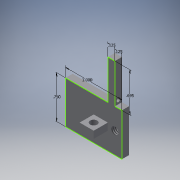
# Autodesk Inventor part: slide pivot plate
Saved by Autodesk Inventor 2016 (Build 200138000, 138)
## iProperties
Created: 2017-01-31
Part Number: slide pivot plate
Material: Generic
Document SubType Name: Modeling
Designer: Mark Koeppen
Density: 1 g/cm^3
Appearance: Default
Mass: 1.61101 g
Surface Area: 14.7029 cm^2
Volume: 1.61101 cm^3
Author: Mark Koeppen
Autodesk Inventor part; units mm, degrees
ref_plane "YZ Plane" through (0, 0, 0) normal (1, 0, 0) x (0, 1, 0)
ref_plane "XZ Plane" through (0, 0, 0) normal (0, 1, 0) x (-1, 0, 0)
ref_plane "XY Plane" through (0, 0, 0) normal (0, 0, 1) x (1, 0, 0)
sketch "Sketch1" plane through (0, 0, 0) normal (0, 0, 1) x (1, 0, 0)
  line L0 (0, -21.016) -> (25.4, -21.016)
  line L1 (25.4, -21.016) -> (25.4, -1.966)
  line L2 (0, -1.966) -> (0, -21.016)
  line L3 (19.05, -1.966) -> (19.05, 15.687)
  line L4 (19.05, 15.687) -> (22.225, 15.687)
  line L5 (22.225, 15.687) -> (22.225, -1.966)
  line L6 (25.4, -1.966) -> (22.225, -1.966)
  line L7 (19.05, -1.966) -> (0, -1.966)
  dimension "d0" = 19.05
  dimension "d2" = 25.4
  dimension "d3" = 3.175
  dimension "d4" = 17.653
  dimension "d22" = 3.175
  constraints: 16 end point, 4 parallel, 4 perpendicular, 1 collinear, 1 horizontal
  measures "d0" distance of L2.start L0.start
  measures "d2" distance of L1.end L2.start
  measures "d3" distance between parallel lines of L5 L3
  measures "d4" distance between parallel lines of L6 L4
  measures "d22" distance between parallel lines of L5 L1
extrude "Extrusion1" add sketch "Sketch1" against normal blind 3.175
sketch "Sketch2" plane through (0, 0, 0) normal (0, 0, 1) x (1, 0, 0)
  line L0 (12.7, -13.0785) -> (19.05, -13.0785)
  line L1 (19.05, -13.0785) -> (19.05, -9.9035)
  line L2 (19.05, -9.9035) -> (12.7, -9.9035)
  line L3 (12.7, -9.9035) -> (12.7, -13.0785)
  line L4 (0, -1.966) -> (0, -21.016) projected
  line L5 (25.4, -1.966) -> (22.225, -1.966) projected
  line L6 (25.4, -21.016) -> (25.4, -1.966) projected
  dimension "d7" = 3.175
  dimension "d10" = 6.35
  dimension "d11" = 7.9375
  dimension "d12" = 6.35
  constraints: 8 end point, 2 parallel, 1 horizontal, 1 perpendicular
  measures "d7" distance between parallel lines of L0 L2
  measures "d10" distance between parallel lines of L1 L3
  measures "d11" distance between parallel lines of L2 L5
  measures "d12" distance between parallel lines of L1 L6
extrude "Extrusion2" add sketch "Sketch2" along normal blind 6.35
sketch "Sketch3" plane through (22.225, -1.966, 0) normal (1, 0, 0) x (0, 0, -1)
  line L0 (0, 0) -> (0, 17.653) projected
  line L1 (0, 0) -> (3.175, 0) projected
  line L2 (3.175, 17.653) -> (3.175, 0) projected
  line L3 (0, 17.653) -> (3.175, 17.653) projected
  point P0 (1.5875, 1.5875)
hole "Hole1" at (22.225, -0.3785, -1.5875) direction (-1, 0, 0) diameter 1.524 end through all
sketch "Sketch4" plane through (12.7, -13.0785, 0) normal (0, -1, 0) x (1, 0, 0)
  line L0 (6.35, 0) -> (0, 0) projected
  line L1 (6.35, 0) -> (6.35, 6.35) projected
  line L2 (0, 6.35) -> (6.35, 6.35) projected
  line L3 (0, 0) -> (0, 6.35) projected
  point P0 (3.175, 3.175)
hole "Hole2" at (15.875, -13.0785, 3.175) direction (0, 1, 0) diameter 3.175 end through all
sketch "Sketch5" plane through (0, 0, -3.175) normal (0, 0, -1) x (-1, 0, 0)
  line L0 (-25.4, -21.016) -> (0, -21.016) projected
  line L1 (0, -21.016) -> (0, -1.966) projected
  line L2 (0, -1.966) -> (-19.05, -1.966) projected
  line L3 (-19.05, -1.966) -> (-19.05, 15.687) projected
  line L4 (-19.05, 15.687) -> (-22.225, 15.687) projected
  line L5 (-22.225, 15.687) -> (-22.225, -1.966) projected
  line L6 (-22.225, -1.966) -> (-25.4, -1.966) projected
  line L7 (-25.4, -1.966) -> (-25.4, -21.016) projected
  point P0 (-22.225, -11.491)
  point P1 (-5.3321, 2.987)
  dimension "d37" = 3.175
  measures "d37" distance from line of point (-22.225, -11.491) L7
hole "Hole3" at (5.3321, 2.987, -3.175) at (22.225, -11.491, -3.175) direction (0, 0, 1) diameter 3.302 end through all thread size "8-32 UNC" class "2B" standard "ANSI Unified Screw Threads"
equation "\"d11\" = -0.5 * d7 + 0.5 * d0"
body "Solid1"
